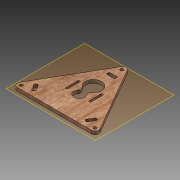
# Autodesk Inventor part: ServoHousingEndPlates
Saved by Autodesk Inventor 2014 SP1 (Build 180222100, 222)
## iProperties
Created: 2014-11-03
Part Number: ServoHousingEndPlates
Material: Wood (Birch)
Document SubType Name: Modeling
Designer: rawrdong
Density: 0.55 g/cm^3
Appearance: Birch - Natural Polished
Author: rawrdong
Autodesk Inventor part; units mm, degrees
ref_plane "YZ Plane" through (0, 0, 0) normal (1, 0, 0) x (0, 1, 0)
ref_plane "XZ Plane" through (0, 0, 0) normal (0, 1, 0) x (-1, 0, 0)
ref_plane "XY Plane" through (0, 0, 0) normal (0, 0, 1) x (1, 0, 0)
ref_plane "Work Plane1" through (0, 0, 0) normal (0, 0, 1) x (1, 0, 0)
sketch "Sketch1" plane through (0, 0, 0) normal (0, 0, 1) x (1, 0, 0)
  circle A0 centre (-34, 58.8897) radius 1.425 projected
  circle A1 centre (-68, 0) radius 1.425 projected
  circle A2 centre (0, 0) radius 1.425 projected
  arc A3 (-2.1152, 2.7886) -> (-3.4725, 0.4375) centre (0, 0) ccw projected
  arc A4 (-3.9686, 0) -> (-3.4725, 0.4375) centre (-3.9686, 0.5) ccw projected
  line L0 (-3.9686, 0) -> (-64.0314, 0) projected
  arc A5 (-64.5275, 0.4375) -> (-64.0314, 0) centre (-64.0314, 0.5) ccw projected
  arc A6 (-64.5275, 0.4375) -> (-65.8848, 2.7886) centre (-68, 0) ccw projected
  arc A7 (-66.0157, 3.4369) -> (-65.8848, 2.7886) centre (-65.5827, 3.1869) ccw projected
  line L1 (-66.0157, 3.4369) -> (-35.9843, 55.4528) projected
  arc A8 (-35.3574, 55.6637) -> (-35.9843, 55.4528) centre (-35.5513, 55.2028) ccw projected
  arc A9 (-35.3574, 55.6637) -> (-32.6426, 55.6637) centre (-34, 58.8897) ccw projected
  arc A10 (-32.0157, 55.4528) -> (-32.6426, 55.6637) centre (-32.4487, 55.2028) ccw projected
  line L2 (-32.0157, 55.4528) -> (-1.9843, 3.4369) projected
  arc A11 (-2.1152, 2.7886) -> (-1.9843, 3.4369) centre (-2.4173, 3.1869) ccw projected
  line L3 (3.0311, 1.75) -> (-30.9689, 60.6397) projected
  arc A12 (-30.9689, 60.6397) -> (-37.0311, 60.6397) centre (-34, 58.8897) ccw projected
  line L4 (-37.0311, 60.6397) -> (-71.0311, 1.75) projected
  arc A13 (-71.0311, 1.75) -> (-68, -3.5) centre (-68, 0) ccw projected
  line L5 (-68, -3.5) -> (0, -3.5) projected
  arc A14 (0, -3.5) -> (3.0311, 1.75) centre (0, 0) ccw projected
  circle A15 centre (-34, 58.8897) radius 1.45
  circle A16 centre (0, 0) radius 1.45
  circle A17 centre (-68, 0) radius 1.45
  line L6 (-59.7303, 1.3104) -> (-62.7303, 6.5066)
  line L7 (-62.3643, 7.8726) -> (-61.4982, 8.3726)
  line L8 (-60.1322, 8.0066) -> (-57.1322, 2.8104)
  line L9 (-57.4982, 1.4444) -> (-58.3643, 0.9444)
  line L10 (-59.2303, 0.4444) -> (-60.6322, 8.8726) construction
  line L11 (-63.2303, 7.3726) -> (-56.6322, 1.9444) construction
  line L12 (-68, 0) -> (-13.9689, 31.1949) construction
  arc A18 (-62.3643, 7.8726) -> (-62.7303, 6.5066) centre (-61.8643, 7.0066) ccw
  arc A19 (-60.1322, 8.0066) -> (-61.4982, 8.3726) centre (-60.9982, 7.5066) ccw
  arc A20 (-57.4982, 1.4444) -> (-57.1322, 2.8104) centre (-57.9982, 2.3104) ccw
  arc A21 (-59.7303, 1.3104) -> (-58.3643, 0.9444) centre (-58.8643, 1.8104) ccw
  line L13 (0, 0) -> (-54.0311, 31.1949) construction
  line L14 (-5.2697, 6.5066) -> (-8.2697, 1.3104)
  line L15 (-9.6357, 0.9444) -> (-10.5018, 1.4444)
  line L16 (-10.8678, 2.8104) -> (-7.8678, 8.0066)
  line L17 (-6.5018, 8.3726) -> (-5.6357, 7.8726)
  line L18 (-4.7697, 7.3726) -> (-11.3678, 1.9444) construction
  line L19 (-8.7697, 0.4444) -> (-7.3678, 8.8726) construction
  line L20 (0, 0) -> (-54.0311, 31.1949) construction
  arc A22 (-9.6357, 0.9444) -> (-8.2697, 1.3104) centre (-9.1357, 1.8104) ccw
  arc A23 (-10.8678, 2.8104) -> (-10.5018, 1.4444) centre (-10.0018, 2.3104) ccw
  arc A24 (-6.5018, 8.3726) -> (-7.8678, 8.0066) centre (-7.0018, 7.5066) ccw
  arc A25 (-5.2697, 6.5066) -> (-5.6357, 7.8726) centre (-6.1357, 7.0066) ccw
  line L21 (-37, 51.0727) -> (-31, 51.0727)
  line L22 (-30, 50.0727) -> (-30, 49.0727)
  line L23 (-31, 48.0727) -> (-37, 48.0727)
  line L24 (-38, 49.0727) -> (-38, 50.0727)
  line L25 (-38, 51.0727) -> (-30, 48.0727) construction
  line L26 (-30, 51.0727) -> (-38, 48.0727) construction
  line L27 (-34, 58.8897) -> (-34, -3.5) construction
  arc A26 (-30, 50.0727) -> (-31, 51.0727) centre (-31, 50.0727) ccw
  arc A27 (-31, 48.0727) -> (-30, 49.0727) centre (-31, 49.0727) ccw
  arc A28 (-38, 49.0727) -> (-37, 48.0727) centre (-37, 49.0727) ccw
  arc A29 (-37, 51.0727) -> (-38, 50.0727) centre (-37, 50.0727) ccw
  point P0 (0, 0)
  point P1 (-59.9312, 4.6585)
  point P2 (-34, 19.6299)
  point P3 (-8.0688, 4.6585)
  point P4 (-34, 19.6299)
  point P5 (-34, 49.5727)
  point P6 (-34, 19.6299)
  dimension "d0" = 2.9
  dimension "d1" = 1
  dimension "d2" = 6
  dimension "d3" = 3
  dimension "d8" = 360
  constraints: 44 end point, 31 point on line, 24 point on circle, 15 centre point, 8 midpoint, 8 tangent, 5 coincident, 5 equal radius, 3 parallel, 1 perpendicular, 92 other
  measures "d0" diameter of A15
  measures "d1" radius of A18
  measures "d2" distance of L8.start L8.end
  measures "d3" distance between parallel lines of L8 L6
extrude "Extrusion1" add sketch "Sketch1" along normal blind 3 contours A3 A4 L0 A5 A6 A7 L1 A8 A9 A10 L2 A11 | A14 L5 A13 L4 A12 L3
sketch "Sketch2" plane through (0, 0, 3) normal (0, 0, 1) x (1, 0, 0)
  line L0 (-37, 51.0727) -> (-31, 51.0727) projected
  line L1 (3.0311, 1.75) -> (-30.9689, 60.6397) projected
  arc A0 (-30.9689, 60.6397) -> (-37.0311, 60.6397) centre (-34, 58.8897) ccw projected
  line L2 (-37.0311, 60.6397) -> (-71.0311, 1.75) projected
  arc A1 (-71.0311, 1.75) -> (-68, -3.5) centre (-68, 0) ccw projected
  arc A2 (0, -3.5) -> (3.0311, 1.75) centre (0, 0) ccw projected
  line L3 (-68, 0) -> (-13.9689, 31.1949) construction
  line L4 (0, 0) -> (-54.0311, 31.1949) construction
  line L5 (-34, 58.8897) -> (-34, -3.4398) construction
  circle A3 centre (-34, 19.6299) radius 5
  line L6 (-43.6292, 30.6595) -> (-45.6292, 30.6595)
  line L7 (-45.6292, 30.6595) -> (-45.6292, 18.1595)
  line L8 (-45.6292, 18.1595) -> (-43.6292, 18.1595)
  line L9 (-43.6292, 18.1595) -> (-43.6292, 30.6595)
  line L10 (-35.468, 24.4095) -> (-53.7034, 24.4095) construction
  line L11 (-24.3708, 30.6595) -> (-22.3708, 30.6595)
  line L12 (-22.3708, 30.6595) -> (-22.3708, 18.1595)
  line L13 (-22.3708, 18.1595) -> (-24.3708, 18.1595)
  line L14 (-24.3708, 18.1595) -> (-24.3708, 30.6595)
  circle A4 centre (-34, 32.6299) radius 7.5
  line L15 (-38.9067, 18.6684) -> (-41.36, 31.1876)
  line L16 (-29.0933, 18.6684) -> (-26.64, 31.1876)
  circle A5 centre (-40.0317, 24.4095) radius 2.6959
  circle A6 centre (-27.9683, 24.4095) radius 2.6959
  point P0 (-29.0016, 19.5045)
  point P1 (-38.9747, 19.1276)
  point P2 (-27.0104, 29.2973)
  point P3 (-37.3373, 23.3531)
  point P4 (-40.9896, 29.2973)
  point P5 (-38.4369, 26.5831)
  point P6 (-37.9188, 22.7352)
  point P7 (-30.0812, 22.7352)
  point P8 (-29.5631, 26.5831)
  dimension "d10" = 10
  dimension "d12" = 12.5
  dimension "d13" = 2
  dimension "d20" = 15
  dimension "d28" = 13
  constraints: 28 end point, 8 point on circle, 8 point on line, 6 symmetric about line, 3 centre point, 3 parallel, 3 tangent, 2 midpoint, 2 perpendicular, 1 coincident, 1 equal radius, 1 horizontal, 14 other
  measures "d12" distance of L11.end L12.end
  measures "d13" distance of L14.end L11.end
  measures "d20" diameter of A4
  measures "d28" distance of A4.centre point (-34, 19.63)
extrude "Extrusion4" cut sketch "Sketch2" against normal through all contours A3 | A5 A4 A6 A3 | A4 | L9 L8 L7 L6 | L11 L12 L13 L14
fillet "Fillet9" radius 1 8 edges at (-45.6292, 30.6595, 1.5) (-43.6292, 30.6595, 1.5) (-45.6292, 18.1595, 1.5) (-43.6292, 18.1595, 1.5) (-24.3708, 18.1595, 1.5) (-22.3708, 18.1595, 1.5) (-24.3708, 30.6595, 1.5) (-22.3708, 30.6595, 1.5)
body "Solid1"
